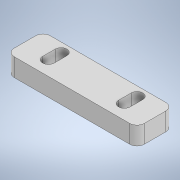
# Autodesk Inventor part: LipoBat Spacer
Saved by Autodesk Inventor 2021 (Build 250183000, 183)
## iProperties
Created: 2020-09-18
Part Number: LipoBat Spacer
Material: Generic
Document SubType Name: Modeling
Designer: jgray
Density: 1 g/cm^3
Appearance: Default
Author: jgray
Autodesk Inventor part; units mm, degrees
ref_plane "YZ Plane" through (0, 0, 0) normal (1, 0, 0) x (0, 1, 0)
ref_plane "XZ Plane" through (0, 0, 0) normal (0, 1, 0) x (-1, 0, 0)
ref_plane "XY Plane" through (0, 0, 0) normal (0, 0, 1) x (1, 0, 0)
sketch "Sketch1" plane through (0, 0, 0) normal (0, 1, 0) x (-1, 0, 0)
  line L0 (0, 0) -> (36, 0)
  line L1 (36, 0) -> (36, -10)
  line L2 (36, -10) -> (0, -10)
  line L3 (0, -10) -> (0, 0)
  line L4 (18, 26.1157) -> (18, -38.8106) construction
  line L5 (28.5, 12.3286) -> (28.5, -24.6324) construction
  line L6 (7.5, 13.3064) -> (7.5, -23.3613) construction
  line L7 (28.5, -7.5) -> (28.5, -4) construction
  line L8 (30.1, -7.5) -> (30.1, -4)
  line L9 (26.9, -4) -> (26.9, -7.5)
  arc A0 (26.9, -7.5) -> (30.1, -7.5) centre (28.5, -7.5) ccw
  arc A1 (30.1, -4) -> (26.9, -4) centre (28.5, -4) ccw
  line L10 (7.5, -7.5) -> (7.5, -4) construction
  line L11 (5.9, -7.5) -> (5.9, -4)
  line L12 (9.1, -4) -> (9.1, -7.5)
  arc A2 (5.9, -7.5) -> (9.1, -7.5) centre (7.5, -7.5) ccw
  arc A3 (9.1, -4) -> (5.9, -4) centre (7.5, -4) ccw
  point P0 (18, 0)
  point P1 (28.5, -5.75)
  point P2 (7.5, -5.75)
  dimension "d0" = 36
  dimension "d1" = 10
  dimension "d2" = 21
  dimension "d3" = 3.5
  dimension "d4" = 3.2
  dimension "d5" = 2.5
  constraints: 30 end point, 8 point on circle, 7 symmetric about line, 4 centre point, 4 tangent, 3 parallel, 3 point on line, 3 vertical, 2 midpoint, 1 horizontal, 1 perpendicular, 3 other
  measures "d0" distance of L1.end L2.end
  measures "d1" distance of L0.end L1.end
  measures "d2" distance between parallel lines of L6 L5
  measures "d3" distance of L7.start L7.end
  measures "d4" diameter of A1
  measures "d5" distance from line of L2 L7.start
extrude "Extrusion1" add sketch "Sketch1" along normal blind 5
fillet "Fillet1" radius 2 4 edges at (0, 2.5, 0) (0, 2.5, -10) (-36, 2.5, -10) (-36, 2.5, 0)
body "Solid1"
